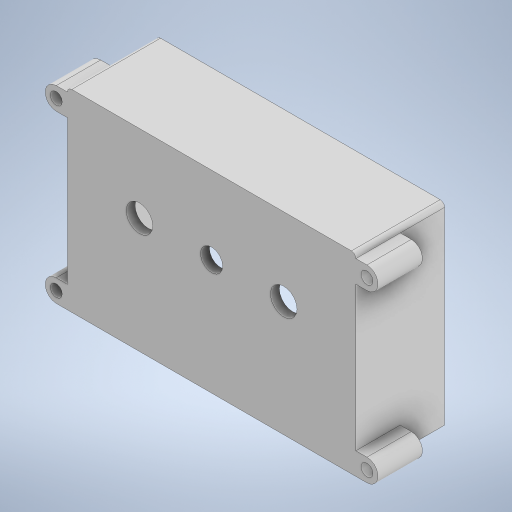
# Autodesk Inventor part: BUTTON COVER
Saved by Autodesk Inventor 2023.1 (Build 271208000, 208)
## iProperties
Created: 2023-02-03
Part Number: BUTTON COVER
Material: Generic
Document SubType Name: Modeling
Designer: liaar
Density: 1 g/cm^3
Appearance: Default
Author: liaar
Autodesk Inventor part; units mm, degrees
ref_plane "YZ Plane" through (0, 0, 0) normal (1, 0, 0) x (0, 1, 0)
ref_plane "XZ Plane" through (0, 0, 0) normal (0, 1, 0) x (-1, 0, 0)
ref_plane "XY Plane" through (0, 0, 0) normal (0, 0, 1) x (1, 0, 0)
sketch "Sketch1" plane through (0, 0, 0) normal (0, 0, 1) x (1, 0, 0)
  line L0 (0, 0) -> (-65, 0)
  line L1 (-65, 0) -> (-65, 43.5)
  line L2 (-65, 43.5) -> (0, 43.5)
  line L3 (0, 43.5) -> (0, 0)
  dimension "d0" = 43.5
  dimension "d1" = 65
  constraints: 8 end point, 2 parallel, 1 horizontal, 1 perpendicular
  measures "d0" distance of L2.end L0.start
  measures "d1" distance of L1.end L2.end
extrude "Extrusion1" add sketch "Sketch1" along normal blind 20
sketch "Sketch2" plane through (0, 0, 0) normal (0, 0, -1) x (-1, 0, 0)
  line L0 (1.8, 41.7) -> (63.2, 41.7)
  line L1 (63.2, 41.7) -> (63.2, 1.8)
  line L2 (63.2, 1.8) -> (1.8, 1.8)
  line L3 (1.8, 1.8) -> (1.8, 41.7)
  line L4 (65, 43.5) -> (65, 0) projected
  line L5 (0, 43.5) -> (65, 43.5) projected
  line L6 (0, 0) -> (0, 43.5) projected
  line L7 (65, 0) -> (0, 0) projected
  point P0 (65, 21.75)
  dimension "d4" = 1.8
  dimension "d5" = 1.8
  dimension "d6" = 1.8
  dimension "d7" = 1.8
  constraints: 8 end point, 2 parallel, 1 horizontal, 1 midpoint, 1 perpendicular
  measures "d4" distance from line of point (65, 21.75) L1
  measures "d5" distance between parallel lines of L5 L0
  measures "d6" distance between parallel lines of L6 L3
  measures "d7" distance between parallel lines of L7 L2
extrude "Extrusion2" cut sketch "Sketch2" against normal blind 18 contours L0 L1 L2 L3
sketch "Sketch3" plane through (0, 0, 20) normal (0, 0, 1) x (1, 0, 0)
  circle A0 centre (-48.75, 26) radius 3
  circle A1 centre (-32.5, 26) radius 2.5
  circle A2 centre (-16.25, 26) radius 3
  line L0 (-65, 43.5) -> (-65, 0) projected
  line L1 (0, 43.5) -> (-65, 43.5) projected
  point P0 (0, 0)
  dimension "d10" = 16.25
  dimension "d11" = 16.25
  dimension "d12" = 16.25
  dimension "d13" = 6
  dimension "d14" = 17.5
  dimension "d15" = 5
  constraints: 3 centre point, 2 horizontal alignment, 1 equal radius
  measures "d10" distance from line of L0 A0.centre
  measures "d11" distance of A1.centre A0.centre
  measures "d12" distance of A1.centre A2.centre
  measures "d13" diameter of A0
  measures "d14" distance from line of L1 A0.centre
  measures "d15" diameter of A1
extrude "Extrusion3" cut sketch "Sketch3" against normal up to surface (2 mm away)
fillet "Fillet1" radius 1 2 edges at (-65, 43.5, 10) (0, 43.5, 10)
sketch "Sketch4" plane through (0, 0, 20) normal (0, 0, 1) x (1, 0, 0)
  line L0 (0, 0) -> (0, 42.5) projected
  line L1 (0, 42.5) -> (5, 42.5)
  line L2 (5, 42.5) -> (5, 37.5)
  line L3 (5, 37.5) -> (0, 37.5)
  line L4 (0, 37.5) -> (0, 42.5)
  line L5 (-65, 42.5) -> (-65, 0) projected
  line L6 (-65, 42.5) -> (-70, 42.5)
  line L7 (-70, 42.5) -> (-70, 37.5)
  line L8 (-70, 37.5) -> (-65, 37.5)
  line L9 (-65, 37.5) -> (-65, 42.5)
  circle A0 centre (-67.5, 40) radius 1.35
  circle A1 centre (2.5, 40) radius 1.35
  line L10 (0, 0) -> (5, 0)
  line L11 (5, 0) -> (5, 5)
  line L12 (5, 5) -> (0, 5)
  line L13 (0, 5) -> (0, 0)
  line L14 (-65, 0) -> (0, 0) projected
  line L15 (-65, 0) -> (-70, 0)
  line L16 (-70, 0) -> (-70, 5)
  line L17 (-70, 5) -> (-65, 5)
  line L18 (-65, 5) -> (-65, 0)
  circle A2 centre (-67.5, 2.5) radius 1.35
  circle A3 centre (2.5, 2.5) radius 1.35
  dimension "d19" = 5
  dimension "d20" = 5
  dimension "d21" = 5
  dimension "d22" = 5
  dimension "d23" = 2.7
  dimension "d24" = 2.7
  dimension "d25" = 5
  dimension "d26" = 5
  dimension "d27" = 5
  dimension "d28" = 5
  dimension "d29" = 2.5
  dimension "d30" = 2.5
  dimension "d31" = 2.5
  dimension "d32" = 2.5
  dimension "d33" = 2.5
  dimension "d34" = 2.5
  dimension "d35" = 2.7
  dimension "d36" = 2.7
  dimension "d37" = 2.5
  dimension "d38" = 2.5
  constraints: 32 end point, 8 parallel, 4 centre point, 4 horizontal, 4 perpendicular
  measures "d19" distance of L5.start L6.end
  measures "d20" distance of L6.end L7.end
  measures "d21" distance of L0.end L1.end
  measures "d22" distance of L1.end L2.end
  measures "d23" diameter of A0
  measures "d24" diameter of A1
  measures "d25" distance of L15.end L16.end
  measures "d26" distance of L5.end L15.end
  measures "d27" distance of L11.end L12.end
  measures "d28" distance of L10.end L11.end
  measures "d29" distance from line of L3 A1.centre
  measures "d30" distance from line of L2 A1.centre
  measures "d31" distance from line of L7 A0.centre
  measures "d32" distance from line of L6 A0.centre
  measures "d33" distance from line of L15 A2.centre
  measures "d34" distance from line of L16 A2.centre
  measures "d35" diameter of A2
  measures "d36" diameter of A3
  measures "d37" distance from line of L0 A3.centre
  measures "d38" distance from line of L12 A3.centre
extrude "Extrusion4" add sketch "Sketch4" against normal blind 10
full round fillet "Full Round Fillet1" first side at (3.3333, 5, 16.6667) centre faces at (5, 1.6667, 16.6667) second side at (-43.3333, 0, 16.6667)
full round fillet "Full Round Fillet2" first side at (-44.1666, 0, 16.6667) centre faces at (-70, 3.3333, 16.6667) second side at (-66.6667, 5, 16.6667)
full round fillet "Full Round Fillet3" first side at (-66.6667, 42.5, 16.6667) centre faces at (-70, 40.8333, 16.6667) second side at (-68.3333, 37.5, 16.6667)
full round fillet "Full Round Fillet4" first side at (1.6667, 37.5, 16.6667) centre faces at (5, 39.1667, 16.6667) second side at (3.3333, 42.5, 16.6667)
body "Solid1"
